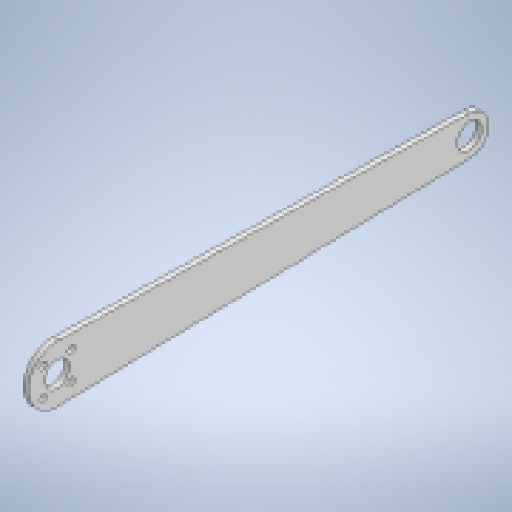
# Autodesk Inventor part: arm
Saved by Autodesk Inventor 2023 (Build 270158000, 158)
## iProperties
Created: 2022-09-10
Part Number: arm
Material: Generic
Document SubType Name: Modeling
Designer: deli
Density: 1 g/cm^3
Appearance: Default
Author: deli
Autodesk Inventor part; units mm, degrees
ref_plane "YZ Plane" through (0, 0, 0) normal (1, 0, 0) x (0, 1, 0)
ref_plane "XZ Plane" through (0, 0, 0) normal (0, 1, 0) x (-1, 0, 0)
ref_plane "XY Plane" through (0, 0, 0) normal (0, 0, 1) x (1, 0, 0)
sketch "Sketch1" plane through (0, 0, 0) normal (1, 0, 0) x (0, 1, 0)
  circle A0 centre (57.6001, -11.8479) radius 2
  circle A1 centre (57.6001, -27.8479) radius 2
  circle A2 centre (41.6001, -27.8479) radius 2
  circle A3 centre (41.6001, -11.8479) radius 2
  line L0 (57.6001, -11.8479) -> (57.6001, -27.8479) construction
  line L1 (57.6001, -27.8479) -> (41.6001, -27.8479) construction
  line L2 (41.6001, -27.8479) -> (41.6001, -11.8479) construction
  line L3 (41.6001, -11.8479) -> (57.6001, -11.8479) construction
  circle A4 centre (49.6001, -19.8479) radius 7
  line L4 (57.6001, -11.8479) -> (41.6001, -27.8479) construction
  line L5 (57.6001, -27.8479) -> (41.6001, -11.8479) construction
  arc A5 (65.5879, -20.4744) -> (33.6039, -20.1928) centre (49.6001, -19.8479) ccw
  circle A6 centre (49.6001, -251.8479) radius 7
  line L6 (49.6001, -19.8479) -> (49.6001, -251.8479) construction
  arc A7 (38.6027, -252.085) -> (60.5976, -252.0849) centre (49.6001, -251.8479) ccw
  line L7 (65.5879, -20.4744) -> (60.5976, -252.0849)
  line L8 (38.6027, -252.085) -> (33.6039, -20.1928)
  point P0 (0, 0)
  dimension "d0" = 4
  dimension "d1" = 4
  dimension "d2" = 4
  dimension "d3" = 4
  dimension "d4" = 16
  dimension "d5" = 16
  dimension "d6" = 14
  dimension "d7" = 32
  dimension "d8" = 14
  dimension "d9" = 232
  dimension "d10" = 4
  constraints: 18 end point, 8 centre point, 4 point on circle, 3 coincident, 3 tangent, 2 perpendicular, 2 vertical, 1 horizontal, 1 midpoint
  measures "d0" diameter of A0
  measures "d1" diameter of A3
  measures "d2" diameter of A2
  measures "d3" diameter of A1
  measures "d4" distance of L0.start L0.end
  measures "d5" distance of L2.end L0.start
  measures "d6" diameter of A4
  measures "d7" diameter of A5
  measures "d8" diameter of A6
  measures "d9" distance of L6.start L6.end
  measures "d10" radial gap between concentric circles of A7 A6
extrude "Extrusion1" add sketch "Sketch1" along normal blind 3.175
equation "\"d1\" = d0"
equation "\"d2\" = d0"
equation "\"d3\" = d0"
body "Solid1"
